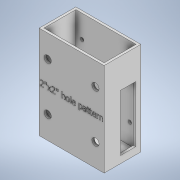
# Autodesk Inventor part: piCaseAttachesToTripodClamp
Saved by Autodesk Inventor 2021.2 (Build 252289000, 289)
## iProperties
Created: 2021-02-07
Part Number: piCaseAttachesToTripodClamp
Material: Generic
Document SubType Name: Modeling
Designer: robst
Density: 1 g/cm^3
Appearance: Default
Author: robst
Autodesk Inventor part; units mm, degrees
ref_plane "YZ Plane" through (0, 0, 0) normal (1, 0, 0) x (0, 1, 0)
ref_plane "XZ Plane" through (0, 0, 0) normal (0, 1, 0) x (-1, 0, 0)
ref_plane "XY Plane" through (0, 0, 0) normal (0, 0, 1) x (1, 0, 0)
sketch "Sketch14" plane through (0, 0, 0) normal (0, 0, 1) x (1, 0, 0)
  line L0 (-34.54, -49.54) -> (34.54, -49.54)
  line L1 (34.54, -49.54) -> (34.54, 49.54)
  line L2 (34.54, 49.54) -> (-34.54, 49.54)
  line L3 (-34.54, 49.54) -> (-34.54, -49.54)
  line L4 (-34.54, -49.54) -> (34.54, 49.54) construction
  line L5 (34.54, -49.54) -> (-34.54, 49.54) construction
  point P0 (0, 0)
  dimension "d66" = 69.08
  dimension "d67" = 99.08
  constraints: 12 end point, 2 midpoint, 2 parallel, 1 horizontal, 1 perpendicular
  measures "d66" distance of L0.start L0.end
  measures "d67" distance of L2.end L0.start
extrude "Extrusion9" add sketch "Sketch14" against normal blind 2.54
sketch "Sketch15" plane through (0, 0, 0) normal (0, 0, 1) x (1, 0, 0)
  line L0 (-34.54, -49.54) -> (-34.54, 49.54) projected
  line L1 (34.54, 49.54) -> (34.54, -49.54) projected
  line L2 (-34.54, -49.54) -> (34.54, -49.54)
  line L3 (34.54, -49.54) -> (34.54, 49.54)
  line L4 (34.54, 49.54) -> (-34.54, 49.54)
  line L5 (-34.54, 49.54) -> (-34.54, -49.54)
  line L6 (-32, -47) -> (32, -47)
  line L7 (32, -47) -> (32, 47)
  line L8 (32, 47) -> (-32, 47)
  line L9 (-32, 47) -> (-32, -47)
  line L10 (-32, -47) -> (32, 47) construction
  line L11 (32, -47) -> (-32, 47) construction
  point P0 (0, 0)
  point P1 (34.54, -49.54)
  dimension "d70" = 64
  dimension "d71" = 94
  constraints: 20 end point, 4 parallel, 2 horizontal, 2 midpoint, 2 perpendicular
  measures "d70" distance of L6.start L6.end
  measures "d71" distance of L8.end L6.start
extrude "Extrusion10" add sketch "Sketch15" along normal blind 34
sketch "Sketch16" plane through (0, 0, 34) normal (0, 0, 1) x (1, 0, 0)
  line L0 (-34.54, -49.54) -> (-34.54, 49.54) projected
  line L1 (34.54, 49.54) -> (34.54, -49.54) projected
  line L2 (-34.54, -49.54) -> (34.54, -49.54)
  line L3 (34.54, -49.54) -> (34.54, 49.54)
  line L4 (34.54, 49.54) -> (-34.54, 49.54)
  line L5 (-34.54, 49.54) -> (-34.54, -49.54)
  point P0 (0, 0)
  point P1 (34.54, -49.54)
  constraints: 8 end point, 2 parallel, 1 horizontal, 1 perpendicular
extrude "Extrusion11" add sketch "Sketch16" along normal blind 2.54
sketch "Sketch17" plane through (-34.54, 49.54, -2.54) normal (0, 1, 0) x (1, 0, 0)
  line L0 (66.54, -2.54) -> (66.54, -36.54) projected
  line L1 (2.54, -36.54) -> (66.54, -36.54) projected
  line L2 (2.54, -2.54) -> (2.54, -36.54) projected
  line L3 (66.54, -2.54) -> (2.54, -2.54) projected
  line L4 (2.54, -36.54) -> (66.54, -36.54)
  line L5 (66.54, -36.54) -> (66.54, -2.54)
  line L6 (66.54, -2.54) -> (2.54, -2.54)
  line L7 (2.54, -2.54) -> (2.54, -36.54)
  point P0 (34.54, -2.54)
  constraints: 8 end point, 2 parallel, 1 horizontal, 1 perpendicular
extrude "Extrusion12" cut sketch "Sketch17" against normal blind 2.54
sketch "Sketch18" plane through (34.54, -49.54, -2.54) normal (1, 0, 0) x (0, 0, -1)
  line L0 (-2.54, 2.54) -> (-2.54, 99.08) projected
  line L1 (-36.54, 99.08) -> (-36.54, 2.54) projected
  line L2 (-2.54, 2.54) -> (-36.54, 2.54) projected
  line L3 (-21.54, 7.54) -> (-5.54, 7.54)
  line L4 (-5.54, 7.54) -> (-5.54, 67.54)
  line L5 (-5.54, 67.54) -> (-21.54, 67.54)
  line L6 (-21.54, 67.54) -> (-21.54, 7.54)
  line L7 (-21.54, 7.54) -> (-5.54, 67.54) construction
  line L8 (-5.54, 7.54) -> (-21.54, 67.54) construction
  line L9 (-39.08, 0) -> (-39.08, 99.08) projected
  point P0 (-2.54, 49.54)
  point P1 (-13.54, 37.54)
  dimension "d78" = 5
  dimension "d79" = 3
  dimension "d80" = 15
  dimension "d81" = 65
  constraints: 12 end point, 2 midpoint, 2 parallel, 2 perpendicular
  measures "d78" distance between parallel lines of L3 L2
  measures "d79" distance between parallel lines of L4 L0
  measures "d80" distance between parallel lines of L6 L1
  measures "d81" distance between parallel lines of L5 L2
extrude "Extrusion13" cut sketch "Sketch18" against normal blind 2.54
sketch "Sketch19" plane through (0, 0, -2.54) normal (0, 0, -1) x (-1, 0, 0)
  line L0 (-25.4, -25.4) -> (25.4, -25.4) construction
  line L1 (25.4, -25.4) -> (25.4, 25.4) construction
  line L2 (25.4, 25.4) -> (-25.4, 25.4) construction
  line L3 (-25.4, 25.4) -> (-25.4, -25.4) construction
  line L4 (-25.4, -25.4) -> (25.4, 25.4) construction
  line L5 (25.4, -25.4) -> (-25.4, 25.4) construction
  point P0 (0, 0)
  dimension "d84" = 50.8
  dimension "d85" = 50.8
  constraints: 12 end point, 2 midpoint, 2 parallel, 1 horizontal, 1 perpendicular
  measures "d84" distance of L0.start L0.end
  measures "d85" distance of L2.end L0.start
hole "Hole3" at (25.4, 25.4, -2.54) at (-25.4, 25.4, -2.54) at (-25.4, -25.4, -2.54) at (25.4, -25.4, -2.54) direction (0, 0, 1) diameter 3.81 end through all clearance for "Flat Head Machine Screw (82)" size "#6" standard "Ansi Unified Screw Threads"
sketch "Sketch22" plane through (0, 0, 36.54) normal (0, 0, 1) x (1, 0, 0)
  circle A0 centre (-25.4, 25.4) radius 1.905 projected
  circle A1 centre (25.4, 25.4) radius 1.905 projected
  circle A2 centre (25.4, -25.4) radius 1.905 projected
  circle A3 centre (-25.4, -25.4) radius 1.905 projected
  point P0 (0, 0)
  constraints: 4 coincident
hole "Hole4" at (-25.4, 25.4, 36.54) at (25.4, 25.4, 36.54) at (25.4, -25.4, 36.54) at (-25.4, -25.4, 36.54) direction (0, 0, -1) diameter 7.62 depth 2.54
sketch "Sketch23" plane through (0, 0, 36.54) normal (0, 0, 1) x (1, 0, 0)
  line L0 (-34.54, 49.54) -> (-34.54, -49.54) construction
  line L1 (-34.54, 0) -> (34.4931, 0) construction
  line L2 (32, -42) -> (32, 18) construction
  line L3 (-29.6044, -3.048) -> (-33.3638, -3.048)
  line L4 (-33.3638, -3.048) -> (-33.3638, -2.1835)
  spline S0 degree 2 poles (-33.3638, -2.1835) (-32.9587, -1.8031) (-32.2374, -1.0967) (-31.8916, -0.7163) knots 0 0 0 1 2 2 2
  spline S1 degree 2 poles (-31.8916, -0.7163) (-31.1951, 0.0494) (-30.6863, 0.9682) (-30.6863, 1.4573) knots 0 0 0 1 2 2 2
  spline S2 degree 2 poles (-30.6863, 1.4573) (-30.6863, 1.7142) (-30.8443, 2.0995) (-30.9876, 2.223) knots 0 0 0 1 2 2 2
  spline S3 degree 2 poles (-30.9876, 2.223) (-31.1309, 2.3465) (-31.5063, 2.47) (-31.7335, 2.47) knots 0 0 0 1 2 2 2
  spline S4 degree 2 poles (-31.7335, 2.47) (-31.9509, 2.47) (-32.3955, 2.3613) (-32.598, 2.2774) knots 0 0 0 1 2 2 2
  spline S5 degree 2 poles (-32.598, 2.2774) (-32.7709, 2.2082) (-33.092, 2.0106) (-33.1909, 1.9414) knots 0 0 0 1 2 2 2
  line L5 (-33.1909, 1.9414) -> (-33.2353, 1.9414)
  line L6 (-33.2353, 1.9414) -> (-33.2353, 2.8109)
  spline S6 degree 2 poles (-33.2353, 2.8109) (-32.9834, 2.9344) (-32.0793, 3.1764) (-31.6743, 3.1764) knots 0 0 0 1 2 2 2
  spline S7 degree 2 poles (-31.6743, 3.1764) (-30.8196, 3.1764) (-29.8563, 2.2724) (-29.8563, 1.5018) knots 0 0 0 1 2 2 2
  spline S8 degree 2 poles (-29.8563, 1.5018) (-29.8563, 1.1411) (-30.0243, 0.5385) (-30.1725, 0.2816) knots 0 0 0 1 2 2 2
  spline S9 degree 2 poles (-30.1725, 0.2816) (-30.3207, 0.0148) (-30.7505, -0.5088) (-30.9876, -0.7608) knots 0 0 0 1 2 2 2
  spline S10 degree 2 poles (-30.9876, -0.7608) (-31.3729, -1.1807) (-32.3165, -2.0798) (-32.598, -2.3416) knots 0 0 0 1 2 2 2
  line L7 (-32.598, -2.3416) -> (-29.6044, -2.3416)
  line L8 (-29.6044, -2.3416) -> (-29.6044, -3.048)
  line L9 (-26.3341, 3.3197) -> (-26.5119, 0.9485)
  line L10 (-26.5119, 0.9485) -> (-27.0504, 0.9485)
  line L11 (-27.0504, 0.9485) -> (-27.2282, 3.3197)
  line L12 (-27.2282, 3.3197) -> (-26.3341, 3.3197)
  line L13 (-27.8754, 3.3197) -> (-28.0532, 0.9485)
  line L14 (-28.0532, 0.9485) -> (-28.5917, 0.9485)
  line L15 (-28.5917, 0.9485) -> (-28.7695, 3.3197)
  line L16 (-28.7695, 3.3197) -> (-27.8754, 3.3197)
  line L17 (-21.7596, -3.048) -> (-22.7032, -3.048)
  line L18 (-22.7032, -3.048) -> (-23.8147, -1.3289)
  line L19 (-23.8147, -1.3289) -> (-24.9558, -3.048)
  line L20 (-24.9558, -3.048) -> (-25.8302, -3.048)
  line L21 (-25.8302, -3.048) -> (-24.2445, -0.7805)
  line L22 (-24.2445, -0.7805) -> (-25.8154, 1.5265)
  line L23 (-25.8154, 1.5265) -> (-24.8718, 1.5265)
  line L24 (-24.8718, 1.5265) -> (-23.7653, -0.1778)
  line L25 (-23.7653, -0.1778) -> (-22.634, 1.5265)
  line L26 (-22.634, 1.5265) -> (-21.7596, 1.5265)
  line L27 (-21.7596, 1.5265) -> (-23.3355, -0.7311)
  line L28 (-23.3355, -0.7311) -> (-21.7596, -3.048)
  line L29 (-17.5161, -3.048) -> (-21.2755, -3.048)
  line L30 (-21.2755, -3.048) -> (-21.2755, -2.1835)
  spline S11 degree 2 poles (-21.2755, -2.1835) (-20.8704, -1.8031) (-20.1492, -1.0967) (-19.8034, -0.7163) knots 0 0 0 1 2 2 2
  spline S12 degree 2 poles (-19.8034, -0.7163) (-19.1068, 0.0494) (-18.598, 0.9682) (-18.598, 1.4573) knots 0 0 0 1 2 2 2
  spline S13 degree 2 poles (-18.598, 1.4573) (-18.598, 1.7142) (-18.7561, 2.0995) (-18.8993, 2.223) knots 0 0 0 1 2 2 2
  spline S14 degree 2 poles (-18.8993, 2.223) (-19.0426, 2.3465) (-19.418, 2.47) (-19.6453, 2.47) knots 0 0 0 1 2 2 2
  spline S15 degree 2 poles (-19.6453, 2.47) (-19.8626, 2.47) (-20.3072, 2.3613) (-20.5098, 2.2774) knots 0 0 0 1 2 2 2
  spline S16 degree 2 poles (-20.5098, 2.2774) (-20.6827, 2.2082) (-21.0038, 2.0106) (-21.1026, 1.9414) knots 0 0 0 1 2 2 2
  line L31 (-21.1026, 1.9414) -> (-21.1471, 1.9414)
  line L32 (-21.1471, 1.9414) -> (-21.1471, 2.8109)
  spline S17 degree 2 poles (-21.1471, 2.8109) (-20.8951, 2.9344) (-19.9911, 3.1764) (-19.586, 3.1764) knots 0 0 0 1 2 2 2
  spline S18 degree 2 poles (-19.586, 3.1764) (-18.7314, 3.1764) (-17.7681, 2.2724) (-17.7681, 1.5018) knots 0 0 0 1 2 2 2
  spline S19 degree 2 poles (-17.7681, 1.5018) (-17.7681, 1.1411) (-17.936, 0.5385) (-18.0842, 0.2816) knots 0 0 0 1 2 2 2
  spline S20 degree 2 poles (-18.0842, 0.2816) (-18.2324, 0.0148) (-18.6622, -0.5088) (-18.8993, -0.7608) knots 0 0 0 1 2 2 2
  spline S21 degree 2 poles (-18.8993, -0.7608) (-19.2847, -1.1807) (-20.2282, -2.0798) (-20.5098, -2.3416) knots 0 0 0 1 2 2 2
  line L33 (-20.5098, -2.3416) -> (-17.5161, -2.3416)
  line L34 (-17.5161, -2.3416) -> (-17.5161, -3.048)
  line L35 (-14.2458, 3.3197) -> (-14.4237, 0.9485)
  line L36 (-14.4237, 0.9485) -> (-14.9621, 0.9485)
  line L37 (-14.9621, 0.9485) -> (-15.14, 3.3197)
  line L38 (-15.14, 3.3197) -> (-14.2458, 3.3197)
  line L39 (-15.7871, 3.3197) -> (-15.965, 0.9485)
  line L40 (-15.965, 0.9485) -> (-16.5034, 0.9485)
  line L41 (-16.5034, 0.9485) -> (-16.6813, 3.3197)
  line L42 (-16.6813, 3.3197) -> (-15.7871, 3.3197)
  line L43 (-7.0136, -3.048) -> (-7.7843, -3.048)
  line L44 (-7.7843, -3.048) -> (-7.7843, -0.4397)
  spline S22 degree 2 poles (-7.7843, -0.4397) (-7.7843, -0.1235) (-7.8435, 0.4199) (-7.9325, 0.5829) knots 0 0 0 1 2 2 2
  spline S23 degree 2 poles (-7.9325, 0.5829) (-8.0263, 0.7558) (-8.3622, 0.9238) (-8.6488, 0.9238) knots 0 0 0 1 2 2 2
  spline S24 degree 2 poles (-8.6488, 0.9238) (-8.9353, 0.9238) (-9.5429, 0.6175) (-9.8344, 0.3705) knots 0 0 0 1 2 2 2
  line L45 (-9.8344, 0.3705) -> (-9.8344, -3.048)
  line L46 (-9.8344, -3.048) -> (-10.605, -3.048)
  line L47 (-10.605, -3.048) -> (-10.605, 3.3197)
  line L48 (-10.605, 3.3197) -> (-9.8344, 3.3197)
  line L49 (-9.8344, 3.3197) -> (-9.8344, 1.0176)
  spline S25 degree 2 poles (-9.8344, 1.0176) (-9.4886, 1.3289) (-8.8217, 1.6549) (-8.4462, 1.6549) knots 0 0 0 1 2 2 2
  spline S26 degree 2 poles (-8.4462, 1.6549) (-7.7744, 1.6549) (-7.0136, 0.7657) (-7.0136, -0.079) knots 0 0 0 1 2 2 2
  line L50 (-7.0136, -0.079) -> (-7.0136, -3.048)
  spline S27 degree 2 poles (-2.1724, -0.7608) (-2.1724, -1.9167) (-3.2839, -3.1764) (-4.2126, -3.1764) knots 0 0 0 1 2 2 2
  spline S28 degree 2 poles (-4.2126, -3.1764) (-5.166, -3.1764) (-6.2578, -1.8772) (-6.2578, -0.7608) knots 0 0 0 1 2 2 2
  spline S29 degree 2 poles (-6.2578, -0.7608) (-6.2578, 0.3853) (-5.1315, 1.6549) (-4.2126, 1.6549) knots 0 0 0 1 2 2 2
  spline S30 degree 2 poles (-4.2126, 1.6549) (-3.2839, 1.6549) (-2.1724, 0.3903) (-2.1724, -0.7608) knots 0 0 0 1 2 2 2
  spline S31 degree 2 poles (-2.9677, -0.7608) (-2.9677, 0.1284) (-3.6149, 0.9929) (-4.2126, 0.9929) knots 0 0 0 1 2 2 2
  spline S32 degree 2 poles (-4.2126, 0.9929) (-4.8104, 0.9929) (-5.4624, 0.1284) (-5.4624, -0.7608) knots 0 0 0 1 2 2 2
  spline S33 degree 2 poles (-5.4624, -0.7608) (-5.4624, -1.6253) (-4.8104, -2.5145) (-4.2126, -2.5145) knots 0 0 0 1 2 2 2
  spline S34 degree 2 poles (-4.2126, -2.5145) (-3.6198, -2.5145) (-2.9677, -1.6401) (-2.9677, -0.7608) knots 0 0 0 1 2 2 2
  line L51 (-0.5965, -3.048) -> (-1.3672, -3.048)
  line L52 (-1.3672, -3.048) -> (-1.3672, 3.3197)
  line L53 (-1.3672, 3.3197) -> (-0.5965, 3.3197)
  line L54 (-0.5965, 3.3197) -> (-0.5965, -3.048)
  spline S35 degree 2 poles (2.5206, -3.1517) (1.424, -3.1517) (0.2186, -1.9217) (0.2186, -0.7855) knots 0 0 0 1 2 2 2
  spline S36 degree 2 poles (0.2186, -0.7855) (0.2186, 0.331) (1.3894, 1.6549) (2.3329, 1.6549) knots 0 0 0 1 2 2 2
  spline S37 degree 2 poles (2.3329, 1.6549) (2.7578, 1.6549) (3.4148, 1.4079) (3.6569, 1.1461) knots 0 0 0 1 2 2 2
  spline S38 degree 2 poles (3.6569, 1.1461) (3.9039, 0.8843) (4.1657, 0.1284) (4.1657, -0.4199) knots 0 0 0 1 2 2 2
  line L55 (4.1657, -0.4199) -> (4.1657, -0.8398)
  line L56 (4.1657, -0.8398) -> (0.9991, -0.8398)
  spline S39 degree 2 poles (0.9991, -0.8398) (0.9991, -1.6352) (1.7994, -2.4799) (2.5108, -2.4799) knots 0 0 0 1 2 2 2
  spline S40 degree 2 poles (2.5108, -2.4799) (2.7627, -2.4799) (3.2518, -2.3663) (3.4494, -2.2774) knots 0 0 0 1 2 2 2
  spline S41 degree 2 poles (3.4494, -2.2774) (3.6569, -2.1786) (3.9434, -2.0057) (4.0372, -1.9266) knots 0 0 0 1 2 2 2
  line L57 (4.0372, -1.9266) -> (4.0817, -1.9266)
  line L58 (4.0817, -1.9266) -> (4.0817, -2.7664)
  spline S42 degree 2 poles (4.0817, -2.7664) (3.9483, -2.8208) (3.5432, -2.9788) (3.3851, -3.0233) knots 0 0 0 1 2 2 2
  spline S43 degree 2 poles (3.3851, -3.0233) (3.1628, -3.0875) (2.7973, -3.1517) (2.5206, -3.1517) knots 0 0 0 1 2 2 2
  spline S44 degree 2 poles (3.4148, -0.2519) (3.4049, 0.0593) (3.2765, 0.5138) (3.153, 0.6669) knots 0 0 0 1 2 2 2
  spline S45 degree 2 poles (3.153, 0.6669) (3.0196, 0.8398) (2.5997, 1.0226) (2.2885, 1.0226) knots 0 0 0 1 2 2 2
  spline S46 degree 2 poles (2.2885, 1.0226) (1.9822, 1.0226) (1.5524, 0.8398) (1.3746, 0.662) knots 0 0 0 1 2 2 2
  spline S47 degree 2 poles (1.3746, 0.662) (1.2017, 0.4792) (1.0238, 0.0395) (0.9991, -0.2519) knots 0 0 0 1 2 2 2
  line L59 (0.9991, -0.2519) -> (3.4148, -0.2519)
  spline S48 degree 2 poles (11.3979, -0.6373) (11.3979, -1.7834) (10.3061, -3.1369) (9.4713, -3.1369) knots 0 0 0 1 2 2 2
  spline S49 degree 2 poles (9.4713, -3.1369) (9.1304, -3.1369) (8.6068, -2.9788) (8.3351, -2.8158) knots 0 0 0 1 2 2 2
  line L60 (8.3351, -2.8158) -> (8.3351, -4.7326)
  line L61 (8.3351, -4.7326) -> (7.5644, -4.7326)
  line L62 (7.5644, -4.7326) -> (7.5644, 1.5265)
  line L63 (7.5644, 1.5265) -> (8.3351, 1.5265)
  line L64 (8.3351, 1.5265) -> (8.3351, 1.0473)
  spline S50 degree 2 poles (8.3351, 1.0473) (8.6216, 1.3091) (9.3231, 1.6549) (9.7331, 1.6549) knots 0 0 0 1 2 2 2
  spline S51 degree 2 poles (9.7331, 1.6549) (10.5186, 1.6549) (11.3979, 0.41) (11.3979, -0.6373) knots 0 0 0 1 2 2 2
  spline S52 degree 2 poles (10.6025, -0.7262) (10.6025, 0.0593) (10.1036, 0.9238) (9.5454, 0.9238) knots 0 0 0 1 2 2 2
  spline S53 degree 2 poles (9.5454, 0.9238) (9.2193, 0.9238) (8.6068, 0.6323) (8.3351, 0.4051) knots 0 0 0 1 2 2 2
  line L65 (8.3351, 0.4051) -> (8.3351, -2.1934)
  spline S54 degree 2 poles (8.3351, -2.1934) (8.6364, -2.3366) (9.0662, -2.4453) (9.3428, -2.4453) knots 0 0 0 1 2 2 2
  spline S55 degree 2 poles (9.3428, -2.4453) (9.9406, -2.4453) (10.6025, -1.566) (10.6025, -0.7262) knots 0 0 0 1 2 2 2
  spline S56 degree 2 poles (14.7472, -2.5639) (14.6534, -2.633) (14.3372, -2.88) (14.189, -2.9541) knots 0 0 0 1 2 2 2
  spline S57 degree 2 poles (14.189, -2.9541) (13.9865, -3.0628) (13.6061, -3.1764) (13.2603, -3.1764) knots 0 0 0 1 2 2 2
  spline S58 degree 2 poles (13.2603, -3.1764) (12.9787, -3.1764) (12.4699, -2.964) (12.2772, -2.7714) knots 0 0 0 1 2 2 2
  spline S59 degree 2 poles (12.2772, -2.7714) (12.0944, -2.5836) (11.8721, -2.0304) (11.8721, -1.7241) knots 0 0 0 1 2 2 2
  spline S60 degree 2 poles (11.8721, -1.7241) (11.8721, -1.2498) (12.2723, -0.578) (12.707, -0.3853) knots 0 0 0 1 2 2 2
  spline S61 degree 2 poles (12.707, -0.3853) (13.0923, -0.2075) (14.1396, -0.0741) (14.7472, -0.0395) knots 0 0 0 1 2 2 2
  line L66 (14.7472, -0.0395) -> (14.7472, 0.1087)
  spline S62 degree 2 poles (14.7472, 0.1087) (14.7472, 0.3754) (14.5842, 0.7064) (14.436, 0.8003) knots 0 0 0 1 2 2 2
  spline S63 degree 2 poles (14.436, 0.8003) (14.2878, 0.8941) (13.863, 0.9534) (13.6357, 0.9534) knots 0 0 0 1 2 2 2
  spline S64 degree 2 poles (13.6357, 0.9534) (13.369, 0.9534) (12.6477, 0.7953) (12.2871, 0.6422) knots 0 0 0 1 2 2 2
  line L67 (12.2871, 0.6422) -> (12.2426, 0.6422)
  line L68 (12.2426, 0.6422) -> (12.2426, 1.4277)
  spline S65 degree 2 poles (12.2426, 1.4277) (12.455, 1.4869) (13.2504, 1.6352) (13.6407, 1.6352) knots 0 0 0 1 2 2 2
  spline S66 degree 2 poles (13.6407, 1.6352) (14.1149, 1.6352) (14.762, 1.4869) (15.0189, 1.2943) knots 0 0 0 1 2 2 2
  spline S67 degree 2 poles (15.0189, 1.2943) (15.2709, 1.1066) (15.5179, 0.5088) (15.5179, 0.079) knots 0 0 0 1 2 2 2
  line L69 (15.5179, 0.079) -> (15.5179, -3.048)
  line L70 (15.5179, -3.048) -> (14.7472, -3.048)
  line L71 (14.7472, -3.048) -> (14.7472, -2.5639)
  line L72 (14.7472, -1.9217) -> (14.7472, -0.6521)
  spline S68 degree 2 poles (14.7472, -0.6521) (14.4706, -0.6768) (13.6357, -0.7608) (13.3739, -0.8398) knots 0 0 0 1 2 2 2
  spline S69 degree 2 poles (13.3739, -0.8398) (13.0676, -0.9337) (12.6675, -1.3239) (12.6675, -1.6697) knots 0 0 0 1 2 2 2
  spline S70 degree 2 poles (12.6675, -1.6697) (12.6675, -2.0649) (13.1121, -2.4651) (13.5369, -2.4651) knots 0 0 0 1 2 2 2
  spline S71 degree 2 poles (13.5369, -2.4651) (13.8975, -2.4651) (14.4903, -2.1539) (14.7472, -1.9217) knots 0 0 0 1 2 2 2
  spline S72 degree 2 poles (17.9829, -3.1369) (17.3556, -3.1369) (16.6491, -2.4206) (16.6491, -1.645) knots 0 0 0 1 2 2 2
  line L73 (16.6491, -1.645) -> (16.6491, 0.8892)
  line L74 (16.6491, 0.8892) -> (16.1304, 0.8892)
  line L75 (16.1304, 0.8892) -> (16.1304, 1.5265)
  line L76 (16.1304, 1.5265) -> (16.6491, 1.5265)
  line L77 (16.6491, 1.5265) -> (16.6491, 2.8405)
  line L78 (16.6491, 2.8405) -> (17.4198, 2.8405)
  line L79 (17.4198, 2.8405) -> (17.4198, 1.5265)
  line L80 (17.4198, 1.5265) -> (18.8376, 1.5265)
  line L81 (18.8376, 1.5265) -> (18.8376, 0.8892)
  line L82 (18.8376, 0.8892) -> (17.4198, 0.8892)
  line L83 (17.4198, 0.8892) -> (17.4198, -1.2893)
  spline S73 degree 2 poles (17.4198, -1.2893) (17.4198, -1.6352) (17.4445, -2.0155) (17.5285, -2.1786) knots 0 0 0 1 2 2 2
  spline S74 degree 2 poles (17.5285, -2.1786) (17.5976, -2.3218) (17.9088, -2.4651) (18.1756, -2.4651) knots 0 0 0 1 2 2 2
  spline S75 degree 2 poles (18.1756, -2.4651) (18.3633, -2.4651) (18.7141, -2.3515) (18.7931, -2.3169) knots 0 0 0 1 2 2 2
  line L84 (18.7931, -2.3169) -> (18.8376, -2.3169)
  line L85 (18.8376, -2.3169) -> (18.8376, -3.0085)
  spline S76 degree 2 poles (18.8376, -3.0085) (18.6202, -3.0678) (18.1756, -3.1369) (17.9829, -3.1369) knots 0 0 0 1 2 2 2
  spline S77 degree 2 poles (20.7889, -3.1369) (20.1615, -3.1369) (19.4551, -2.4206) (19.4551, -1.645) knots 0 0 0 1 2 2 2
  line L86 (19.4551, -1.645) -> (19.4551, 0.8892)
  line L87 (19.4551, 0.8892) -> (18.9364, 0.8892)
  line L88 (18.9364, 0.8892) -> (18.9364, 1.5265)
  line L89 (18.9364, 1.5265) -> (19.4551, 1.5265)
  line L90 (19.4551, 1.5265) -> (19.4551, 2.8405)
  line L91 (19.4551, 2.8405) -> (20.2257, 2.8405)
  line L92 (20.2257, 2.8405) -> (20.2257, 1.5265)
  line L93 (20.2257, 1.5265) -> (21.6435, 1.5265)
  line L94 (21.6435, 1.5265) -> (21.6435, 0.8892)
  line L95 (21.6435, 0.8892) -> (20.2257, 0.8892)
  line L96 (20.2257, 0.8892) -> (20.2257, -1.2893)
  spline S78 degree 2 poles (20.2257, -1.2893) (20.2257, -1.6352) (20.2504, -2.0155) (20.3344, -2.1786) knots 0 0 0 1 2 2 2
  spline S79 degree 2 poles (20.3344, -2.1786) (20.4036, -2.3218) (20.7148, -2.4651) (20.9815, -2.4651) knots 0 0 0 1 2 2 2
  spline S80 degree 2 poles (20.9815, -2.4651) (21.1693, -2.4651) (21.52, -2.3515) (21.599, -2.3169) knots 0 0 0 1 2 2 2
  line L97 (21.599, -2.3169) -> (21.6435, -2.3169)
  line L98 (21.6435, -2.3169) -> (21.6435, -3.0085)
  spline S81 degree 2 poles (21.6435, -3.0085) (21.4261, -3.0678) (20.9815, -3.1369) (20.7889, -3.1369) knots 0 0 0 1 2 2 2
  spline S82 degree 2 poles (24.1975, -3.1517) (23.1008, -3.1517) (21.8955, -1.9217) (21.8955, -0.7855) knots 0 0 0 1 2 2 2
  spline S83 degree 2 poles (21.8955, -0.7855) (21.8955, 0.331) (23.0662, 1.6549) (24.0098, 1.6549) knots 0 0 0 1 2 2 2
  spline S84 degree 2 poles (24.0098, 1.6549) (24.4346, 1.6549) (25.0917, 1.4079) (25.3337, 1.1461) knots 0 0 0 1 2 2 2
  spline S85 degree 2 poles (25.3337, 1.1461) (25.5807, 0.8843) (25.8425, 0.1284) (25.8425, -0.4199) knots 0 0 0 1 2 2 2
  line L99 (25.8425, -0.4199) -> (25.8425, -0.8398)
  line L100 (25.8425, -0.8398) -> (22.676, -0.8398)
  spline S86 degree 2 poles (22.676, -0.8398) (22.676, -1.6352) (23.4763, -2.4799) (24.1876, -2.4799) knots 0 0 0 1 2 2 2
  spline S87 degree 2 poles (24.1876, -2.4799) (24.4396, -2.4799) (24.9286, -2.3663) (25.1262, -2.2774) knots 0 0 0 1 2 2 2
  spline S88 degree 2 poles (25.1262, -2.2774) (25.3337, -2.1786) (25.6202, -2.0057) (25.7141, -1.9266) knots 0 0 0 1 2 2 2
  line L101 (25.7141, -1.9266) -> (25.7586, -1.9266)
  line L102 (25.7586, -1.9266) -> (25.7586, -2.7664)
  spline S89 degree 2 poles (25.7586, -2.7664) (25.6252, -2.8208) (25.2201, -2.9788) (25.062, -3.0233) knots 0 0 0 1 2 2 2
  spline S90 degree 2 poles (25.062, -3.0233) (24.8397, -3.0875) (24.4741, -3.1517) (24.1975, -3.1517) knots 0 0 0 1 2 2 2
  spline S91 degree 2 poles (25.0917, -0.2519) (25.0818, 0.0593) (24.9533, 0.5138) (24.8298, 0.6669) knots 0 0 0 1 2 2 2
  spline S92 degree 2 poles (24.8298, 0.6669) (24.6964, 0.8398) (24.2765, 1.0226) (23.9653, 1.0226) knots 0 0 0 1 2 2 2
  spline S93 degree 2 poles (23.9653, 1.0226) (23.659, 1.0226) (23.2293, 0.8398) (23.0514, 0.662) knots 0 0 0 1 2 2 2
  spline S94 degree 2 poles (23.0514, 0.662) (22.8785, 0.4792) (22.7007, 0.0395) (22.676, -0.2519) knots 0 0 0 1 2 2 2
  line L103 (22.676, -0.2519) -> (25.0917, -0.2519)
  line L104 (29.0486, 0.7015) -> (29.0091, 0.7015)
  spline S95 degree 2 poles (29.0091, 0.7015) (28.9202, 0.7262) (28.7275, 0.7361) (28.5941, 0.7361) knots 0 0 0 1 2 2 2
  spline S96 degree 2 poles (28.5941, 0.7361) (28.2829, 0.7361) (27.6703, 0.4644) (27.3937, 0.1976) knots 0 0 0 1 2 2 2
  line L105 (27.3937, 0.1976) -> (27.3937, -3.048)
  line L106 (27.3937, -3.048) -> (26.6231, -3.048)
  line L107 (26.6231, -3.048) -> (26.6231, 1.5265)
  line L108 (26.6231, 1.5265) -> (27.3937, 1.5265)
  line L109 (27.3937, 1.5265) -> (27.3937, 0.8447)
  spline S97 degree 2 poles (27.3937, 0.8447) (27.8136, 1.2202) (28.441, 1.5265) (28.7374, 1.5265) knots 0 0 0 1 2 2 2
  spline S98 degree 2 poles (28.7374, 1.5265) (28.856, 1.5265) (28.9745, 1.5166) (29.0486, 1.5018) knots 0 0 0 1 2 2 2
  line L110 (29.0486, 1.5018) -> (29.0486, 0.7015)
  line L111 (33.2378, -3.048) -> (32.4671, -3.048)
  line L112 (32.4671, -3.048) -> (32.4671, -0.4397)
  spline S99 degree 2 poles (32.4671, -0.4397) (32.4671, -0.1235) (32.4078, 0.4199) (32.3189, 0.5829) knots 0 0 0 1 2 2 2
  spline S100 degree 2 poles (32.3189, 0.5829) (32.2251, 0.7558) (31.8891, 0.9238) (31.6026, 0.9238) knots 0 0 0 1 2 2 2
  spline S101 degree 2 poles (31.6026, 0.9238) (31.3161, 0.9238) (30.7085, 0.6175) (30.417, 0.3705) knots 0 0 0 1 2 2 2
  line L113 (30.417, 0.3705) -> (30.417, -3.048)
  line L114 (30.417, -3.048) -> (29.6464, -3.048)
  line L115 (29.6464, -3.048) -> (29.6464, 1.5265)
  line L116 (29.6464, 1.5265) -> (30.417, 1.5265)
  line L117 (30.417, 1.5265) -> (30.417, 1.0176)
  spline S102 degree 2 poles (30.417, 1.0176) (30.7628, 1.3289) (31.4297, 1.6549) (31.8052, 1.6549) knots 0 0 0 1 2 2 2
  spline S103 degree 2 poles (31.8052, 1.6549) (32.477, 1.6549) (33.2378, 0.7657) (33.2378, -0.079) knots 0 0 0 1 2 2 2
  line L118 (33.2378, -0.079) -> (33.2378, -3.048)
  point P0 (0, 0)
  constraints: 2 end point, 1 horizontal, 1 midpoint, 1 perpendicular
extrude "Extrusion14" cut sketch "Sketch23" against normal blind 1.27
equation "\"d66\" = piBoxExteriorWidth"
equation "\"d67\" = piBoxExteriorLength"
equation "\"d68\" = piBoxWallThickness"
equation "\"d70\" = piBoxInteriorWidth"
equation "\"d71\" = piBoxInteriorLength"
equation "\"d72\" = piBoxInteriorHeight"
equation "\"d74\" = piBoxWallThickness"
equation "\"d76\" = piBoxWallThickness"
equation "\"d82\" = piBoxWallThickness"
equation "\"piBoxInteriorLength\" = 94"
equation "\"piBoxInteriorWidth\" = 64"
equation "\"piBoxInteriorHeight\" = 34"
equation "\"piBoxThickness\" = 3.175"
equation "\"piBoxWallThickness\" = 2.54"
equation "\"piBoxExteriorLength\" = piBoxInteriorLength + 2 * piBoxWallThickness"
equation "\"piBoxExteriorHeight\" = piBoxInteriorHeight + piBoxWallThickness"
equation "\"piBoxExteriorWidth\" = piBoxInteriorWidth + 2 * piBoxWallThickness"
body "Solid1"
body "Solid2"
